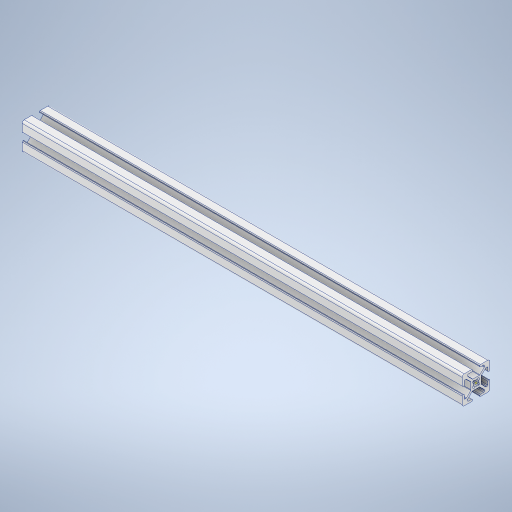
# Autodesk Inventor part: 2020_400
Saved by Autodesk Inventor 2024 (Build 280153000, 153)
## iProperties
Created: 2025-12-15
Part Number: 2020_400
Material: Aluminum 6061
Document SubType Name: Modeling
Designer: schar
Density: 2.7 g/cm^3
Appearance: Aluminum - Flat
Author: schar
Autodesk Inventor part; units mm, degrees
ref_plane "YZ Plane" through (0, 0, 0) normal (1, 0, 0) x (0, 1, 0)
ref_plane "XZ Plane" through (0, 0, 0) normal (0, 1, 0) x (-1, 0, 0)
ref_plane "XY Plane" through (0, 0, 0) normal (0, 0, 1) x (1, 0, 0)
sketch "Sketch1" plane through (0, 0, 0) normal (1, 0, 0) x (0, 1, 0)
  arc A0 (0.804, -1.9351) -> (2.1249, -2.3045) centre (1.5684, -1.748) ccw
  line L0 (2.1249, -2.3045) -> (2.3045, -2.1249)
  arc A1 (2.3045, -2.1249) -> (1.9351, -0.804) centre (1.748, -1.5684) ccw
  arc A2 (1.9351, -0.804) -> (1.9351, 0.804) centre (0, 0) ccw
  arc A3 (1.9351, 0.804) -> (2.3045, 2.1249) centre (1.748, 1.5684) ccw
  line L1 (2.3045, 2.1249) -> (2.1249, 2.3045)
  arc A4 (2.1249, 2.3045) -> (0.804, 1.9351) centre (1.5684, 1.748) ccw
  arc A5 (0.804, 1.9351) -> (-0.804, 1.9351) centre (0, 0) ccw
  arc A6 (-0.804, 1.9351) -> (-2.1249, 2.3045) centre (-1.5684, 1.748) ccw
  line L2 (-2.1249, 2.3045) -> (-2.3045, 2.1249)
  arc A7 (-2.3045, 2.1249) -> (-1.9351, 0.804) centre (-1.748, 1.5684) ccw
  arc A8 (-1.9351, 0.804) -> (-1.9351, -0.804) centre (0, 0) ccw
  arc A9 (-1.9351, -0.804) -> (-2.3045, -2.1249) centre (-1.748, -1.5684) ccw
  line L3 (-2.3045, -2.1249) -> (-2.1249, -2.3045)
  arc A10 (-2.1249, -2.3045) -> (-0.804, -1.9351) centre (-1.5684, -1.748) ccw
  arc A11 (-0.804, -1.9351) -> (0.804, -1.9351) centre (0, 0) ccw
  line L4 (9.008, 2.63) -> (9.492, 2.63)
  arc A12 (8.5, 3.138) -> (9.008, 2.63) centre (9.008, 3.138) ccw
  line L5 (8.5, 5.487) -> (8.5, 3.138)
  arc A13 (8.5, 5.487) -> (7.992, 5.995) centre (7.992, 5.487) ccw
  line L6 (7.2661, 5.995) -> (7.992, 5.995)
  arc A14 (7.2661, 5.995) -> (6.9069, 5.8462) centre (7.2661, 5.487) ccw
  line L7 (3.8038, 2.7431) -> (6.9069, 5.8462)
  arc A15 (3.8038, 2.7431) -> (3.655, 2.3839) centre (4.163, 2.3839) ccw
  line L8 (3.655, -2.3839) -> (3.655, 2.3839)
  arc A16 (3.655, -2.3839) -> (3.8038, -2.7431) centre (4.163, -2.3839) ccw
  line L9 (6.9069, -5.8462) -> (3.8038, -2.7431)
  arc A17 (6.9069, -5.8462) -> (7.2661, -5.995) centre (7.2661, -5.487) ccw
  line L10 (7.992, -5.995) -> (7.2661, -5.995)
  arc A18 (7.992, -5.995) -> (8.5, -5.487) centre (7.992, -5.487) ccw
  line L11 (8.5, -3.138) -> (8.5, -5.487)
  arc A19 (9.008, -2.63) -> (8.5, -3.138) centre (9.008, -3.138) ccw
  line L12 (9.492, -2.63) -> (9.008, -2.63)
  arc A20 (10, -3.138) -> (9.492, -2.63) centre (9.492, -3.138) ccw
  line L13 (10, -8.5) -> (10, -3.138)
  arc A21 (8.5, -10) -> (10, -8.5) centre (8.5, -8.5) ccw
  line L14 (3.138, -10) -> (8.5, -10)
  arc A22 (2.63, -9.492) -> (3.138, -10) centre (3.138, -9.492) ccw
  line L15 (2.63, -9.008) -> (2.63, -9.492)
  arc A23 (3.138, -8.5) -> (2.63, -9.008) centre (3.138, -9.008) ccw
  line L16 (5.487, -8.5) -> (3.138, -8.5)
  arc A24 (5.487, -8.5) -> (5.995, -7.992) centre (5.487, -7.992) ccw
  line L17 (5.995, -7.2661) -> (5.995, -7.992)
  arc A25 (5.995, -7.2661) -> (5.8462, -6.9069) centre (5.487, -7.2661) ccw
  line L18 (2.7431, -3.8038) -> (5.8462, -6.9069)
  arc A26 (2.7431, -3.8038) -> (2.3839, -3.655) centre (2.3839, -4.163) ccw
  line L19 (-2.3839, -3.655) -> (2.3839, -3.655)
  arc A27 (-2.3839, -3.655) -> (-2.7431, -3.8038) centre (-2.3839, -4.163) ccw
  line L20 (-5.8462, -6.9069) -> (-2.7431, -3.8038)
  arc A28 (-5.8462, -6.9069) -> (-5.995, -7.2661) centre (-5.487, -7.2661) ccw
  line L21 (-5.995, -7.992) -> (-5.995, -7.2661)
  arc A29 (-5.995, -7.992) -> (-5.487, -8.5) centre (-5.487, -7.992) ccw
  line L22 (-3.138, -8.5) -> (-5.487, -8.5)
  arc A30 (-2.63, -9.008) -> (-3.138, -8.5) centre (-3.138, -9.008) ccw
  line L23 (-2.63, -9.492) -> (-2.63, -9.008)
  arc A31 (-3.138, -10) -> (-2.63, -9.492) centre (-3.138, -9.492) ccw
  line L24 (-8.5, -10) -> (-3.138, -10)
  arc A32 (-10, -8.5) -> (-8.5, -10) centre (-8.5, -8.5) ccw
  line L25 (-10, -3.138) -> (-10, -8.5)
  arc A33 (-9.492, -2.63) -> (-10, -3.138) centre (-9.492, -3.138) ccw
  line L26 (-9.008, -2.63) -> (-9.492, -2.63)
  arc A34 (-8.5, -3.138) -> (-9.008, -2.63) centre (-9.008, -3.138) ccw
  line L27 (-8.5, -5.487) -> (-8.5, -3.138)
  arc A35 (-8.5, -5.487) -> (-7.992, -5.995) centre (-7.992, -5.487) ccw
  line L28 (-7.2661, -5.995) -> (-7.992, -5.995)
  arc A36 (-7.2661, -5.995) -> (-6.9069, -5.8462) centre (-7.2661, -5.487) ccw
  line L29 (-3.8038, -2.7431) -> (-6.9069, -5.8462)
  arc A37 (-3.8038, -2.7431) -> (-3.655, -2.3839) centre (-4.163, -2.3839) ccw
  line L30 (-3.655, 2.3839) -> (-3.655, -2.3839)
  arc A38 (-3.655, 2.3839) -> (-3.8038, 2.7431) centre (-4.163, 2.3839) ccw
  line L31 (-6.9069, 5.8462) -> (-3.8038, 2.7431)
  arc A39 (-6.9069, 5.8462) -> (-7.2661, 5.995) centre (-7.2661, 5.487) ccw
  line L32 (-7.992, 5.995) -> (-7.2661, 5.995)
  arc A40 (-7.992, 5.995) -> (-8.5, 5.487) centre (-7.992, 5.487) ccw
  line L33 (-8.5, 3.138) -> (-8.5, 5.487)
  arc A41 (-9.008, 2.63) -> (-8.5, 3.138) centre (-9.008, 3.138) ccw
  line L34 (-9.492, 2.63) -> (-9.008, 2.63)
  arc A42 (-10, 3.138) -> (-9.492, 2.63) centre (-9.492, 3.138) ccw
  line L35 (-10, 8.5) -> (-10, 3.138)
  arc A43 (-8.5, 10) -> (-10, 8.5) centre (-8.5, 8.5) ccw
  line L36 (-3.138, 10) -> (-8.5, 10)
  arc A44 (-2.63, 9.492) -> (-3.138, 10) centre (-3.138, 9.492) ccw
  line L37 (-2.63, 9.008) -> (-2.63, 9.492)
  arc A45 (-3.138, 8.5) -> (-2.63, 9.008) centre (-3.138, 9.008) ccw
  line L38 (-5.487, 8.5) -> (-3.138, 8.5)
  arc A46 (-5.487, 8.5) -> (-5.995, 7.992) centre (-5.487, 7.992) ccw
  line L39 (-5.995, 7.2661) -> (-5.995, 7.992)
  arc A47 (-5.995, 7.2661) -> (-5.8462, 6.9069) centre (-5.487, 7.2661) ccw
  line L40 (-2.7431, 3.8038) -> (-5.8462, 6.9069)
  arc A48 (-2.7431, 3.8038) -> (-2.3839, 3.655) centre (-2.3839, 4.163) ccw
  line L41 (2.3839, 3.655) -> (-2.3839, 3.655)
  arc A49 (2.3839, 3.655) -> (2.7431, 3.8038) centre (2.3839, 4.163) ccw
  line L42 (5.8462, 6.9069) -> (2.7431, 3.8038)
  arc A50 (5.8462, 6.9069) -> (5.995, 7.2661) centre (5.487, 7.2661) ccw
  line L43 (5.995, 7.992) -> (5.995, 7.2661)
  arc A51 (5.995, 7.992) -> (5.487, 8.5) centre (5.487, 7.992) ccw
  line L44 (3.138, 8.5) -> (5.487, 8.5)
  arc A52 (2.63, 9.008) -> (3.138, 8.5) centre (3.138, 9.008) ccw
  line L45 (2.63, 9.492) -> (2.63, 9.008)
  arc A53 (3.138, 10) -> (2.63, 9.492) centre (3.138, 9.492) ccw
  line L46 (8.5, 10) -> (3.138, 10)
  arc A54 (10, 8.5) -> (8.5, 10) centre (8.5, 8.5) ccw
  line L47 (10, 3.138) -> (10, 8.5)
  arc A55 (9.492, 2.63) -> (10, 3.138) centre (9.492, 3.138) ccw
  point P0 (0.804, -1.9351)
  point P1 (-0.804, -1.9351)
  point P2 (-2.3045, -2.1249)
  point P3 (-1.9351, -0.804)
  point P4 (-1.9351, 0.804)
  point P5 (-2.1249, 2.3045)
  point P6 (-0.804, 1.9351)
  point P7 (0.804, 1.9351)
  point P8 (2.3045, 2.1249)
  point P9 (1.9351, 0.804)
  point P10 (1.9351, -0.804)
  point P11 (2.1249, -2.3045)
  point P12 (8.5, 3.138)
  point P13 (10, 8.5)
  point P14 (3.138, 10)
  point P15 (2.63, 9.008)
  point P16 (5.487, 8.5)
  point P17 (5.995, 7.2661)
  point P18 (2.7431, 3.8038)
  point P19 (-2.3839, 3.655)
  point P20 (-5.8462, 6.9069)
  point P21 (-5.995, 7.992)
  point P22 (-3.138, 8.5)
  point P23 (-2.63, 9.492)
  point P24 (-8.5, 10)
  point P25 (-10, 3.138)
  point P26 (-9.008, 2.63)
  point P27 (-8.5, 5.487)
  point P28 (-7.2661, 5.995)
  point P29 (-3.8038, 2.7431)
  point P30 (-3.655, -2.3839)
  point P31 (-6.9069, -5.8462)
  point P32 (-7.992, -5.995)
  point P33 (-8.5, -3.138)
  point P34 (-9.492, -2.63)
  point P35 (-10, -8.5)
  point P36 (-3.138, -10)
  point P37 (-2.63, -9.008)
  point P38 (-5.487, -8.5)
  point P39 (-5.995, -7.2661)
  point P40 (-2.7431, -3.8038)
  point P41 (2.3839, -3.655)
  point P42 (5.8462, -6.9069)
  point P43 (5.995, -7.992)
  point P44 (3.138, -8.5)
  point P45 (2.63, -9.492)
  point P46 (8.5, -10)
  point P47 (10, -3.138)
  point P48 (9.008, -2.63)
  point P49 (8.5, -5.487)
  point P50 (7.2661, -5.995)
  point P51 (3.8038, -2.7431)
  point P52 (3.655, 2.3839)
  point P53 (6.9069, 5.8462)
  point P54 (7.992, 5.995)
  constraints: 112 point on circle, 96 end point, 56 centre point
extrude "Extrusion1" add sketch "Sketch1" along normal blind 380
sketch "Sketch2" plane through (0, 3.138, 10) normal (0, 0, 1) x (1, 0, 0)
  line L0 (0, -3.138) -> (15, -3.138)
  circle A0 centre (15, -3.138) radius 2.5
  circle A1 centre (53, -3.138) radius 2.5
  circle A2 centre (91, -3.138) radius 2.5
  dimension "d2" = 15
  dimension "d3" = 5
  dimension "d6" = 38
  constraints: 3 centre point, 2 end point, 2 horizontal, 1 coincident, 4 other
  measures "d2" distance of L0.start L0.end
  measures "d3" diameter of A0
  measures "d6" distance of A0.centre A1.centre
extrude "Extrusion2" cut sketch "Sketch2" against normal blind 400
sketch "Sketch3" plane through (380, 0, 0) normal (1, 0, 0) x (0, 0, -1)
  line L0 (-14.0219, 14.4978) -> (24.7854, 14.4978)
  line L1 (24.7854, 14.4978) -> (24.7854, -18.1589)
  line L2 (24.7854, -18.1589) -> (-14.0219, -18.1589)
  line L3 (-14.0219, -18.1589) -> (-14.0219, 14.4978)
  point P0 (0, 0)
  constraints: 8 end point, 2 parallel, 1 horizontal, 1 perpendicular
extrude "Extrusion3" cut sketch "Sketch3" against normal blind 62.711
sketch "Sketch4" plane through (0, 8.5, 10) normal (0, 0, 1) x (1, 0, 0)
  line L0 (317.289, 0.508) -> (317.289, 0) projected
  line L1 (317.289, 0) -> (317.289, -8.5)
  line L2 (317.289, -6.1161) -> (317.289, -10.8839) projected
  line L3 (317.289, -8.5) -> (307.289, -8.5)
  circle A0 centre (307.289, -8.5) radius 2
  point P0 (0, -8.5)
  dimension "d15" = 10
  dimension "d16" = 4
  constraints: 4 end point, 1 centre point, 1 coincident, 1 horizontal, 1 midpoint
  measures "d15" distance of L1.end L3.end
  measures "d16" diameter of A0
extrude "Extrusion4" cut sketch "Sketch4" against normal through all
sketch "Sketch5" plane through (317.289, 0, 0) normal (1, 0, 0) x (0, 0, -1)
  point P0 (0, 0)
body "Solid1"
